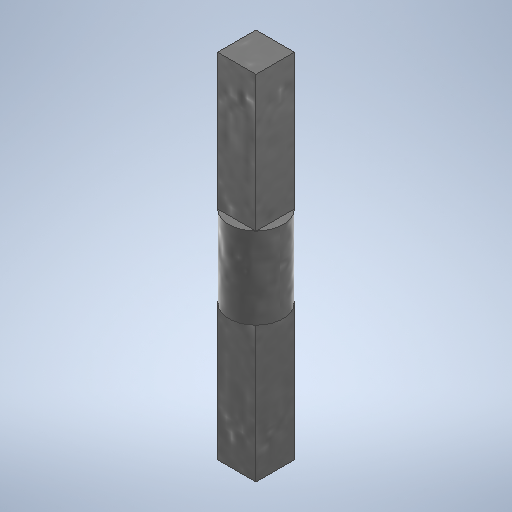
# Autodesk Inventor part: SCARA swivel connection rod
Saved by Autodesk Inventor 2025.2 (Build 292293000, 293)
## iProperties
Created: 2025-01-26
Part Number: SCARA swivel connection rod
Material: Generic
Document SubType Name: Modeling
Designer: caomi
Density: 1 g/cm^3
Appearance: Default
Author: caomi
Autodesk Inventor part; units mm, degrees
ref_plane "YZ Plane" through (0, 0, 0) normal (1, 0, 0) x (0, 1, 0)
ref_plane "XZ Plane" through (0, 0, 0) normal (0, 1, 0) x (-1, 0, 0)
ref_plane "XY Plane" through (0, 0, 0) normal (0, 0, 1) x (1, 0, 0)
sketch "Sketch1" plane through (0, 0, 0) normal (0, 1, 0) x (-1, 0, 0)
  circle A0 centre (0, 0) radius 4
  dimension "d0" = 8
  constraints: 1 centre point, 1 coincident
  measures "d0" diameter of A0
extrude "Extrusion1" add sketch "Sketch1" along normal blind 12
sketch "Sketch2" plane through (0, 12, 0) normal (0, 1, 0) x (1, 0, 0)
  line L0 (2.8284, 2.8284) -> (-2.8284, 2.8284)
  line L1 (-2.8284, 2.8284) -> (-2.8284, -2.8284)
  line L2 (-2.8284, -2.8284) -> (2.8284, -2.8284)
  line L3 (2.8284, -2.8284) -> (2.8284, 2.8284)
  line L4 (2.8284, 2.8284) -> (-2.8284, -2.8284) construction
  line L5 (-2.8284, 2.8284) -> (2.8284, -2.8284) construction
  circle A0 centre (0, 0) radius 4 projected
  constraints: 12 end point, 2 midpoint, 2 parallel, 2 perpendicular, 1 horizontal, 2 other
extrude "Extrusion2" add sketch "Sketch2" along normal blind 20 contours L3 L2 L1 L0
sketch "Sketch3" plane through (0, 0, 0) normal (0, -1, 0) x (1, 0, 0)
  line L0 (2.8284, -2.8284) -> (-2.8284, -2.8284)
  line L1 (-2.8284, -2.8284) -> (-2.8284, 2.8284)
  line L2 (-2.8284, 2.8284) -> (2.8284, 2.8284)
  line L3 (2.8284, 2.8284) -> (2.8284, -2.8284)
  line L4 (2.8284, -2.8284) -> (-2.8284, 2.8284) construction
  line L5 (-2.8284, -2.8284) -> (2.8284, 2.8284) construction
  circle A0 centre (0, 0) radius 4 projected
  constraints: 12 end point, 2 midpoint, 2 parallel, 2 perpendicular, 1 horizontal, 2 other
extrude "Extrusion3" add sketch "Sketch3" along normal blind 20 contours L0 L1 L2 L3
body "Solid1"
